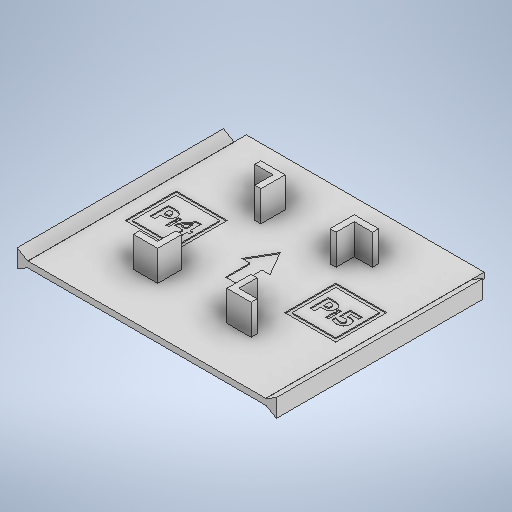
# Autodesk Inventor part: Suelo
Saved by Autodesk Inventor 2025.1 (Build 291241000, 241)
## iProperties
Created: 2025-11-20
Part Number: Suelo
Material: Genérico
Document SubType Name: Modeling
Designer: Diego
Density: 1 g/cm^3
Appearance: Valor por defecto
Author: Diego
Autodesk Inventor part; units mm, degrees
sketch "Boceto1" plane through (0, 0, 0) normal (0, 0, 1) x (1, 0, 0)
  line L0 (-107.4375, 9.96) -> (-116.4375, 15.1562) construction
  line L1 (-116.4375, 15.1562) -> (-116.4375, -0.2361) construction
  line L2 (-116.4375, -0.2361) -> (-107.4375, 4.96) construction
  line L3 (-107.4375, 9.96) -> (-98.4042, 9.96) construction
  line L4 (-107.4375, 4.96) -> (-97.9616, 4.96) construction
  line L5 (-107.4375, 12.46) -> (-107.4375, 9.96) construction
  line L6 (-107.4375, 12.46) -> (-107.4375, 9.96) construction
  line L7 (-107.4375, 5.1333) -> (-115.5375, 0.4567)
  line L8 (-107.4375, 9.7868) -> (-115.5375, 14.4634)
  line L9 (-116.2875, 0.8897) -> (-116.2875, 14.0304)
  line L10 (-107.4375, 9.96) -> (-107.4375, 4.96) construction
  line L11 (-107.4375, 7.46) -> (88.5625, 7.46) construction
  line L12 (-9.4375, 45.8997) -> (-9.4375, -33.2811) construction
  line L13 (-107.4375, 9.7868) -> (-107.4375, 5.1333)
  line L14 (88.5625, 4.96) -> (79.0866, 4.96) construction
  line L15 (88.5625, 9.96) -> (79.5293, 9.96) construction
  line L16 (88.5625, 12.46) -> (88.5625, 9.96) construction
  line L17 (88.5625, 12.46) -> (88.5625, 9.96) construction
  line L18 (97.5625, 15.1562) -> (97.5625, -0.2361) construction
  line L19 (97.5625, -0.2361) -> (88.5625, 4.96) construction
  line L20 (88.5625, 9.96) -> (97.5625, 15.1562) construction
  line L21 (88.5625, 5.1333) -> (96.6625, 0.4567)
  line L22 (88.5625, 9.7868) -> (96.6625, 14.4634)
  line L23 (97.4125, 0.8897) -> (97.4125, 14.0304)
  line L24 (88.5625, 9.96) -> (88.5625, 4.96) construction
  line L25 (88.5625, 9.7868) -> (88.5625, 5.1333)
  line L26 (96.6625, 14.4634) -> (97.4125, 14.8964)
  line L27 (97.4125, 14.8964) -> (97.4125, 14.0304)
  line L28 (96.6625, 0.4567) -> (97.4125, 0.0237)
  line L29 (97.4125, 0.0237) -> (97.4125, 0.8897)
  line L30 (-116.2875, 14.0304) -> (-116.2875, 14.8964)
  line L31 (-115.5375, 14.4634) -> (-116.2875, 14.8964)
  line L32 (-116.2875, 0.8897) -> (-116.2875, 0.0237)
  line L33 (-115.5375, 0.4567) -> (-116.2875, 0.0237)
  point P0 (0, 0)
  point P1 (-116.4375, 7.46)
  point P2 (-111.9375, 12.5581)
  point P3 (-9.4375, 7.46)
  point P4 (97.5625, 7.46)
  point P5 (93.0625, 12.5581)
  dimension "d0" = 60
  dimension "d49" = 0.15
  dimension "d51" = 0.15
  constraints: 68 end point, 13 point on line, 13 symmetric about line, 10 vertical, 4 midpoint, 3 horizontal, 3 parallel, 1 collinear, 2 other
  measures "d0" angle of L0 L1
  measures "d49" distance between parallel lines of L2 L7
  measures "d51" distance between parallel lines of L0 L8
ref_plane "Plano de trabajo4" through (0, 0, 0) normal (0, 0, 1) x (1, 0, 0)
sketch "Boceto2" plane through (0, 0, 0) normal (0, 0, 1) x (1, 0, 0)
  line L0 (-107.4375, 9.96) -> (-107.4375, 4.96) projected
  line L1 (97.5625, -0.2361) -> (88.5625, 4.96) projected
  line L2 (-107.4375, 9.96) -> (88.5625, 9.96)
  line L3 (88.5625, 9.96) -> (88.5625, 4.96)
  line L4 (88.5625, 4.96) -> (-107.4375, 4.96)
  line L5 (-107.4375, 4.96) -> (-107.4375, 9.96)
  point P0 (0, 0)
  constraints: 8 end point, 2 parallel, 1 horizontal, 1 perpendicular
extrude "Extrusión2" add sketch "Boceto2" against normal blind 180
ref_plane "Plano de trabajo2" through (-107.4375, 9.96, 0) normal (0, 1, 0) x (1, 0, 0)
sketch "Boceto3" plane through (-107.4375, 9.96, 0) normal (0, 1, 0) x (1, 0, 0)
  line L0 (0, 0) -> (196, 0) projected
  line L1 (0, 0) -> (0, 170) projected
  line L2 (0, 180) -> (64.5, 180) construction
  line L3 (64.5, 180) -> (64.5, 42.5) construction
  line L4 (64.5, 42.5) -> (0, 42.5) construction
  line L5 (0, 42.5) -> (0, 180) construction
  line L6 (0, 180) -> (196, 180) projected
  line L7 (0, 170) -> (0, 180) projected
  line L8 (196, 180) -> (0, 180) construction
  line L9 (98, 180) -> (98, 0) construction
  line L10 (64.5, 90) -> (0, 90) construction
  line L11 (32.25, 180) -> (32.25, 42.5) construction
  line L12 (64.5, 108) -> (0, 108) construction
  line L13 (64.5, 72) -> (0, 72) construction
  line L14 (64.5, 42.5) -> (64.5, 57.5)
  line L15 (64.5, 57.5) -> (69.5, 57.5)
  line L16 (69.5, 57.5) -> (69.5, 37.5)
  line L17 (69.5, 37.5) -> (49.5, 37.5)
  line L18 (49.5, 37.5) -> (49.5, 42.5)
  line L19 (49.5, 42.5) -> (64.5, 42.5)
  line L20 (64.5, 137.5) -> (64.5, 122.5)
  line L21 (64.5, 122.5) -> (69.5, 122.5)
  line L22 (69.5, 122.5) -> (69.5, 142.5)
  line L23 (69.5, 142.5) -> (49.5, 142.5)
  line L24 (49.5, 142.5) -> (49.5, 137.5)
  line L25 (49.5, 137.5) -> (64.5, 137.5)
  line L26 (131.5, 42.5) -> (131.5, 57.5)
  line L27 (131.5, 57.5) -> (126.5, 57.5)
  line L28 (126.5, 57.5) -> (126.5, 37.5)
  line L29 (126.5, 37.5) -> (146.5, 37.5)
  line L30 (146.5, 37.5) -> (146.5, 42.5)
  line L31 (146.5, 42.5) -> (131.5, 42.5)
  line L32 (131.5, 122.5) -> (126.5, 122.5)
  line L33 (131.5, 137.5) -> (131.5, 122.5)
  line L34 (146.5, 137.5) -> (131.5, 137.5)
  line L35 (126.5, 122.5) -> (126.5, 142.5)
  line L36 (146.5, 142.5) -> (146.5, 137.5)
  line L37 (126.5, 142.5) -> (146.5, 142.5)
  point P0 (107.4375, 0)
  point P1 (32.25, 137.5)
  point P2 (131.5, 90)
  point P3 (131.5, 108)
  point P4 (131.5, 72)
  dimension "d14" = 36
  dimension "d21" = 37.5
  dimension "d22" = 5
  dimension "d23" = 20
  dimension "d24" = 5
  dimension "d25" = 64.5
  dimension "d26" = 20
  dimension "d27" = 47.5
  constraints: 66 end point, 22 symmetric about line, 10 point on line, 8 perpendicular, 4 midpoint, 2 horizontal, 2 parallel, 1 other
  measures "d14" distance between parallel lines of L13 L12
  measures "d21" distance between parallel lines of L0 L17
  measures "d22" distance of L17.end L18.end
  measures "d23" distance of L16.end L17.end
  measures "d24" distance of L14.end L15.end
  measures "d25" distance between parallel lines of L1 L14
  measures "d26" distance of L15.end L16.end
  measures "d27" distance between parallel lines of L19 L10
ref_plane "Plano de trabajo3" through (-107.4375, 9.96, 0) normal (0, 1, 0) x (1, 0, 0)
sketch "Boceto4" plane through (-107.4375, 9.96, 0) normal (0, 1, 0) x (1, 0, 0)
  line L0 (12.9564, 124.5347) -> (51.5436, 124.5347) construction
  line L1 (51.5436, 124.5347) -> (51.5436, 55.4653) construction
  line L2 (51.5436, 55.4653) -> (12.9564, 55.4653) construction
  line L3 (12.9564, 55.4653) -> (12.9564, 124.5347) construction
  line L4 (64.5, 108) -> (0, 108) construction
  line L5 (64.5, 90) -> (0, 90) construction
  line L6 (64.5, 72) -> (0, 72) construction
  line L7 (64.5, 180) -> (64.5, 42.5) construction
  line L8 (32.25, 180) -> (32.25, 42.5) construction
  line L9 (98, 180) -> (98, 0) construction
  line L10 (131.5, 108) -> (196, 108) construction
  line L11 (131.5, 90) -> (196, 90) construction
  line L12 (131.5, 72) -> (196, 72) construction
  line L13 (163.75, 180) -> (163.75, 42.5) construction
  line L14 (131.5, 180) -> (131.5, 42.5) construction
  line L15 (14.25, 72) -> (50.25, 72)
  line L16 (50.25, 72) -> (50.25, 108)
  line L17 (50.25, 108) -> (14.25, 108)
  line L18 (14.25, 108) -> (14.25, 72)
  line L19 (14.25, 72) -> (50.25, 108) construction
  line L20 (50.25, 72) -> (14.25, 108) construction
  line L21 (11.25, 69) -> (53.25, 69)
  line L22 (53.25, 69) -> (53.25, 111)
  line L23 (53.25, 111) -> (11.25, 111)
  line L24 (11.25, 111) -> (11.25, 69)
  line L25 (181.75, 72) -> (145.75, 72)
  line L26 (145.75, 72) -> (145.75, 108)
  line L27 (145.75, 108) -> (181.75, 108)
  line L28 (181.75, 108) -> (181.75, 72)
  line L29 (181.75, 72) -> (145.75, 108) construction
  line L30 (145.75, 72) -> (181.75, 108) construction
  line L31 (184.75, 69) -> (142.75, 69)
  line L32 (142.75, 69) -> (142.75, 111)
  line L33 (142.75, 111) -> (184.75, 111)
  line L34 (184.75, 111) -> (184.75, 69)
  line L35 (93, 90) -> (93, 70)
  line L36 (93, 70) -> (103, 70)
  line L37 (103, 70) -> (103, 90)
  line L38 (103, 90) -> (93, 70) construction
  line L39 (93, 90) -> (103, 70) construction
  line L40 (93, 90) -> (86.453, 90)
  line L41 (86.453, 90) -> (98, 110)
  line L42 (98, 110) -> (109.547, 90)
  line L43 (109.547, 90) -> (103, 90)
  line L44 (196, 0) -> (0, 0) projected
  line L45 (152.3173, 101.4327) -> (175.1827, 101.4327) construction
  line L46 (175.1827, 101.4327) -> (175.1827, 78.5673) construction
  line L47 (175.1827, 78.5673) -> (152.3173, 78.5673) construction
  line L48 (152.3173, 78.5673) -> (152.3173, 101.4327) construction
  spline S0 degree 2 poles (29.9202, 92.7897) (29.9202, 91.7443) (29.2516, 89.8481) (28.6317, 89.216) knots 0 0 0 1 2 2 2
  spline S1 degree 2 poles (28.6317, 89.216) (28.2549, 88.8148) (27.331, 88.1584) (26.784, 87.9275) knots 0 0 0 1 2 2 2
  spline S2 degree 2 poles (26.784, 87.9275) (26.2249, 87.6965) (24.9242, 87.4291) (24.122, 87.4291) knots 0 0 0 1 2 2 2
  line L49 (24.122, 87.4291) -> (22.1528, 87.4291)
  line L50 (22.1528, 87.4291) -> (22.1528, 82.5182)
  line L51 (22.1528, 82.5182) -> (18.3845, 82.5182)
  line L52 (18.3845, 82.5182) -> (18.3845, 97.5182)
  line L53 (18.3845, 97.5182) -> (24.2071, 97.5182)
  spline S3 degree 2 poles (24.2071, 97.5182) (25.4955, 97.5182) (27.3797, 97.0442) (28.1455, 96.5336) knots 0 0 0 1 2 2 2
  spline S4 degree 2 poles (28.1455, 96.5336) (28.9964, 95.9623) (29.9202, 94.0904) (29.9202, 92.7897) knots 0 0 0 1 2 2 2
  spline S5 degree 2 poles (26.0547, 92.6925) (26.0547, 93.3367) (25.4469, 94.2484) (25.0336, 94.4186) knots 0 0 0 1 2 2 2
  spline S6 degree 2 poles (25.0336, 94.4186) (24.4988, 94.6495) (23.5263, 94.7224) (22.6876, 94.7224) knots 0 0 0 1 2 2 2
  line L54 (22.6876, 94.7224) -> (22.1528, 94.7224)
  line L55 (22.1528, 94.7224) -> (22.1528, 90.2249)
  line L56 (22.1528, 90.2249) -> (22.4202, 90.2249)
  spline S7 degree 2 poles (22.4202, 90.2249) (22.9429, 90.2249) (23.891, 90.2492) (24.2435, 90.31) knots 0 0 0 1 2 2 2
  spline S8 degree 2 poles (24.2435, 90.31) (24.5474, 90.3586) (25.216, 90.6503) (25.3983, 90.8327) knots 0 0 0 1 2 2 2
  spline S9 degree 2 poles (25.3983, 90.8327) (25.7873, 91.1973) (26.0547, 92.0118) (26.0547, 92.6925) knots 0 0 0 1 2 2 2
  line L57 (33.6317, 82.5182) -> (31.2816, 82.5182)
  line L58 (31.2816, 82.5182) -> (31.2816, 90.0628)
  line L59 (31.2816, 90.0628) -> (33.6317, 90.0628)
  line L60 (33.6317, 90.0628) -> (33.6317, 82.5182)
  line L61 (33.7046, 91.1406) -> (31.2168, 91.1406)
  line L62 (31.2168, 91.1406) -> (31.2168, 92.972)
  line L63 (31.2168, 92.972) -> (33.7046, 92.972)
  line L64 (33.7046, 92.972) -> (33.7046, 91.1406)
  line L65 (47.2581, 86.019) -> (45.2281, 86.019)
  line L66 (45.2281, 86.019) -> (45.2281, 82.4818)
  line L67 (45.2281, 82.4818) -> (41.5936, 82.4818)
  line L68 (41.5936, 82.4818) -> (41.5936, 86.019)
  line L69 (41.5936, 86.019) -> (34.981, 86.019)
  line L70 (34.981, 86.019) -> (34.981, 88.8148)
  line L71 (34.981, 88.8148) -> (41.472, 97.5182)
  line L72 (41.472, 97.5182) -> (45.2281, 97.5182)
  line L73 (45.2281, 97.5182) -> (45.2281, 88.7176)
  line L74 (45.2281, 88.7176) -> (47.2581, 88.7176)
  line L75 (47.2581, 88.7176) -> (47.2581, 86.019)
  line L76 (41.5936, 88.7176) -> (41.5936, 93.8229)
  line L77 (41.5936, 93.8229) -> (37.7889, 88.7176)
  line L78 (37.7889, 88.7176) -> (41.5936, 88.7176)
  spline S10 degree 2 poles (161.4202, 92.9295) (161.4202, 91.8841) (160.7516, 89.9878) (160.1317, 89.3558) knots 0 0 0 1 2 2 2
  spline S11 degree 2 poles (160.1317, 89.3558) (159.7549, 88.9546) (158.831, 88.2982) (158.284, 88.0673) knots 0 0 0 1 2 2 2
  spline S12 degree 2 poles (158.284, 88.0673) (157.7249, 87.8363) (156.4242, 87.5689) (155.622, 87.5689) knots 0 0 0 1 2 2 2
  line L79 (155.622, 87.5689) -> (153.6528, 87.5689)
  line L80 (153.6528, 87.5689) -> (153.6528, 82.658)
  line L81 (153.6528, 82.658) -> (149.8845, 82.658)
  line L82 (149.8845, 82.658) -> (149.8845, 97.658)
  line L83 (149.8845, 97.658) -> (155.7071, 97.658)
  spline S13 degree 2 poles (155.7071, 97.658) (156.9955, 97.658) (158.8797, 97.184) (159.6455, 96.6734) knots 0 0 0 1 2 2 2
  spline S14 degree 2 poles (159.6455, 96.6734) (160.4964, 96.1021) (161.4202, 94.2301) (161.4202, 92.9295) knots 0 0 0 1 2 2 2
  spline S15 degree 2 poles (157.5547, 92.8323) (157.5547, 93.4765) (156.9469, 94.3882) (156.5336, 94.5583) knots 0 0 0 1 2 2 2
  spline S16 degree 2 poles (156.5336, 94.5583) (155.9988, 94.7893) (155.0263, 94.8622) (154.1876, 94.8622) knots 0 0 0 1 2 2 2
  line L84 (154.1876, 94.8622) -> (153.6528, 94.8622)
  line L85 (153.6528, 94.8622) -> (153.6528, 90.3647)
  line L86 (153.6528, 90.3647) -> (153.9202, 90.3647)
  spline S17 degree 2 poles (153.9202, 90.3647) (154.4429, 90.3647) (155.391, 90.389) (155.7435, 90.4498) knots 0 0 0 1 2 2 2
  spline S18 degree 2 poles (155.7435, 90.4498) (156.0474, 90.4984) (156.716, 90.7901) (156.8983, 90.9724) knots 0 0 0 1 2 2 2
  spline S19 degree 2 poles (156.8983, 90.9724) (157.2873, 91.3371) (157.5547, 92.1515) (157.5547, 92.8323) knots 0 0 0 1 2 2 2
  line L87 (165.1317, 82.658) -> (162.7816, 82.658)
  line L88 (162.7816, 82.658) -> (162.7816, 90.2026)
  line L89 (162.7816, 90.2026) -> (165.1317, 90.2026)
  line L90 (165.1317, 90.2026) -> (165.1317, 82.658)
  line L91 (165.2046, 91.2804) -> (162.7168, 91.2804)
  line L92 (162.7168, 91.2804) -> (162.7168, 93.1118)
  line L93 (162.7168, 93.1118) -> (165.2046, 93.1118)
  line L94 (165.2046, 93.1118) -> (165.2046, 91.2804)
  spline S20 degree 2 poles (178.2354, 87.7391) (178.2354, 86.56) (177.4331, 84.5665) (176.643, 83.8493) knots 0 0 0 1 2 2 2
  spline S21 degree 2 poles (176.643, 83.8493) (175.8529, 83.1321) (173.6892, 82.342) (172.109, 82.342) knots 0 0 0 1 2 2 2
  spline S22 degree 2 poles (172.109, 82.342) (170.4315, 82.3541) (168.0247, 82.9011) (167.2346, 83.2536) knots 0 0 0 1 2 2 2
  line L95 (167.2346, 83.2536) -> (167.2346, 86.5235)
  line L96 (167.2346, 86.5235) -> (167.575, 86.5235)
  spline S23 degree 2 poles (167.575, 86.5235) (167.8667, 86.3655) (168.5717, 85.9522) (169.143, 85.7334) knots 0 0 0 1 2 2 2
  spline S24 degree 2 poles (169.143, 85.7334) (169.6779, 85.5267) (170.784, 85.2472) (171.4526, 85.2472) knots 0 0 0 1 2 2 2
  spline S25 degree 2 poles (171.4526, 85.2472) (172.0361, 85.2472) (173.3975, 85.5389) (173.8108, 85.9279) knots 0 0 0 1 2 2 2
  spline S26 degree 2 poles (173.8108, 85.9279) (174.1147, 86.2318) (174.455, 86.9733) (174.455, 87.5932) knots 0 0 0 1 2 2 2
  spline S27 degree 2 poles (174.455, 87.5932) (174.455, 88.128) (174.0174, 88.8817) (173.6649, 89.1126) knots 0 0 0 1 2 2 2
  spline S28 degree 2 poles (173.6649, 89.1126) (173.1544, 89.453) (171.6957, 89.6475) (171.173, 89.6475) knots 0 0 0 1 2 2 2
  spline S29 degree 2 poles (171.173, 89.6475) (170.3464, 89.6475) (168.7784, 89.3801) (168.2071, 89.2342) knots 0 0 0 1 2 2 2
  line L97 (168.2071, 89.2342) -> (167.8788, 89.2342)
  line L98 (167.8788, 89.2342) -> (167.8788, 97.658)
  line L99 (167.8788, 97.658) -> (177.8221, 97.658)
  line L100 (177.8221, 97.658) -> (177.8221, 94.8258)
  line L101 (177.8221, 94.8258) -> (171.4404, 94.8258)
  line L102 (171.4404, 94.8258) -> (171.4404, 92.3339)
  spline S30 degree 2 poles (171.4404, 92.3339) (171.7443, 92.3582) (172.5831, 92.3825) (172.814, 92.3825) knots 0 0 0 1 2 2 2
  spline S31 degree 2 poles (172.814, 92.3825) (173.8959, 92.3825) (175.7192, 91.9449) (176.4364, 91.4951) knots 0 0 0 1 2 2 2
  spline S32 degree 2 poles (176.4364, 91.4951) (177.2873, 90.936) (178.2354, 89.0762) (178.2354, 87.7391) knots 0 0 0 1 2 2 2
  point P0 (107.4375, 0)
  point P1 (32.25, 90)
  point P2 (163.75, 90)
  point P3 (98, 80)
  dimension "d15" = 36
  dimension "d16" = 36
  dimension "d17" = 3
  dimension "d30" = 10
  dimension "d31" = 20
  dimension "d33" = 60
  dimension "d34" = 60
  dimension "d35" = 60
  dimension "d37" = 20
  dimension "d38" = 90
  constraints: 68 end point, 19 symmetric about line, 6 equal length, 5 midpoint, 5 point on line, 3 horizontal, 2 perpendicular, 2 vertical, 11 other
  measures "d15" distance of L17.end L16.end
  measures "d16" distance of L15.end L16.end
  measures "d17" distance between parallel lines of L18 L24
  measures "d30" distance of L35.end L36.end
  measures "d31" distance of L36.end L37.end
  measures "d33" angle of L40 L41
  measures "d34" angle of L43 L42
  measures "d35" angle of L42 L41
  measures "d37" distance from line of L43 L41.end
  measures "d38" distance between parallel lines of L44 L40
extrude "Extrusión3" add sketch "Boceto3" along normal blind 25
extrude "Extrusión5" cut sketch "Boceto4" against normal blind 0.8
extrude "Extrusión6" add sketch "Boceto1" against normal blind 170
equation "\"d3\" = L_base"
equation "\"d14\" = Font"
equation "\"d16\" = d15"
equation "\"L_base\" = 180"
equation "\"W_Pi\" = 64.5"
equation "\"L_Pi\" = 95"
equation "\"Font\" = 36"
